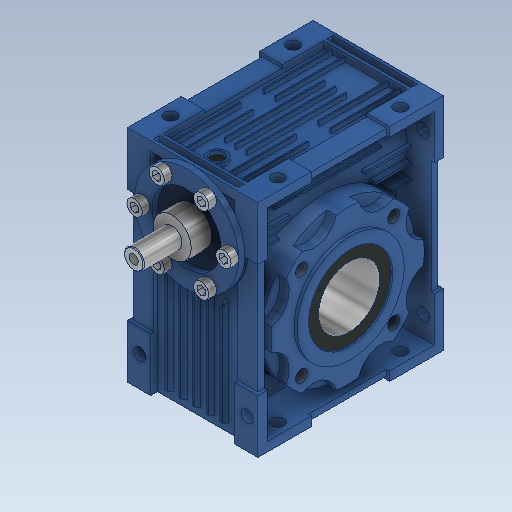
# Autodesk Inventor part: nmrv 50 casing
Saved by Autodesk Inventor 2020 (Build 240168000, 168)
## iProperties
Created: 2020-07-31
Part Number: nmrv 50 casing
Material: Generic
Document SubType Name: Modeling
Designer: Vikki
Density: 3.52796 g/cm^3
Appearance: Flaked Satin - Blue
Mass: 3500 g
Surface Area: 1630.31 cm^2
Volume: 992.076 cm^3
Author: Vikki
Autodesk Inventor part; units mm, degrees
sketch "Sketch1" plane through (0, 0, 0) normal (1, 0, 0) x (0, 1, 0)
  line L0 (-72, 60.5) -> (72, 60.5)
  line L1 (72, 60.5) -> (72, -60.5)
  line L2 (72, -60.5) -> (-72, -60.5)
  line L3 (-72, -60.5) -> (-72, 60.5)
  line L4 (-72, 60.5) -> (72, -60.5) construction
  line L5 (72, 60.5) -> (-72, -60.5) construction
  circle A0 centre (0, 0) radius 20
  dimension "d0" = 144
  dimension "d1" = 121
  dimension "d2" = 40
  constraints: 12 end point, 2 parallel, 1 centre point, 1 horizontal, 1 perpendicular, 1 vertical
  measures "d0" distance of L1.end L2.end
  measures "d1" distance of L0.end L1.end
  measures "d2" diameter of A0
extrude "Extrusion1" add sketch "Sketch1" along normal blind 85
ref_plane "Work Plane4" through (72.5, 0, 0) normal (1, 0, 0) x (0, 0, -1)
ref_plane "Work Plane5" through (85, 0, 0) normal (1, 0, 0) x (0, 0, -1)
sketch "Sketch10" plane through (0, 72, 60.5) normal (0, 1, 0) x (1, 0, 0)
  line L0 (0, 121) -> (0, 0) projected
  line L1 (0, 0) -> (85, 0) projected
  line L2 (85, 121) -> (85, 0) projected
  line L3 (0, 121) -> (85, 121) projected
  line L4 (0, 121) -> (0, 0) projected
  line L5 (0, 121) -> (85, 121) projected
  line L6 (0, 0) -> (85, 121)
  line L7 (0, 121) -> (85, 0)
  line L8 (77.5, 20.5) -> (7.5, 20.5)
  line L9 (7.5, 20.5) -> (7.5, 100.5)
  line L10 (7.5, 100.5) -> (77.5, 100.5)
  line L11 (77.5, 100.5) -> (77.5, 20.5)
  line L12 (77.5, 20.5) -> (7.5, 100.5) construction
  line L13 (7.5, 20.5) -> (77.5, 100.5) construction
  circle A0 centre (7.5, 20.5) radius 4.1
  circle A1 centre (7.5, 100.5) radius 4.1
  circle A2 centre (77.5, 100.5) radius 4.1
  circle A3 centre (77.5, 20.5) radius 4.1
  point P0 (0, 60.5)
  point P1 (42.5, 60.5)
  dimension "d60" = 70
  dimension "d61" = 80
  dimension "d62" = 8.2
  constraints: 16 end point, 4 centre point, 4 coincident, 3 equal radius, 3 midpoint, 2 parallel, 1 horizontal, 1 perpendicular
  measures "d60" distance of L9.end L10.end
  measures "d61" distance of L8.end L9.end
  measures "d62" diameter of A0
extrude "Extrusion10" cut sketch "Sketch10" against normal blind 10 contours A1 L9 L10 | L10 L9 A1 | A0 L9 L8 | L8 L9 A0 | A2 L11 L10 | L10 L11 A2 | A3 L11 L8 | L8 L11 A3
ref_plane "Work Plane6" through (0, 57, 60.5) normal (0, -1, 0) x (1, 0, 0)
sketch "Sketch14" plane through (0, 72, 60.5) normal (0, 1, 0) x (1, 0, 0)
  line L0 (0, 0) -> (85, 0) projected
  line L1 (0, 121) -> (85, 121) projected
  line L2 (0, 0) -> (85, 121)
  line L3 (0, 121) -> (0, 0) projected
  line L4 (0, 121) -> (85, 0)
  line L5 (70, -9.5) -> (15, -9.5)
  line L6 (15, -9.5) -> (15, 130.5)
  line L7 (15, 130.5) -> (70, 130.5)
  line L8 (70, 130.5) -> (70, -9.5)
  line L9 (70, -9.5) -> (15, 130.5) construction
  line L10 (15, -9.5) -> (70, 130.5) construction
  point P0 (0, 60.5)
  point P1 (42.5, 60.5)
  dimension "d74" = 140
  dimension "d75" = 55
  constraints: 16 end point, 3 midpoint, 2 parallel, 1 horizontal, 1 perpendicular
  measures "d74" distance of L5.end L6.end
  measures "d75" distance of L6.end L7.end
extrude "Extrusion13" cut sketch "Sketch14" against normal blind 5 contours L6 L2 L4 L8 L0 | L0 L8 L5 L6 | L6 L4 L2 | L4 L6 L1 L8 L2 | L2 L8 L4 | L6 L7 L8 L1
sketch "Sketch15" plane through (0, 67, 60.5) normal (0, 1, 0) x (1, 0, 0)
  line L0 (15, 0) -> (70, 0)
  line L1 (70, 0) -> (70, 2)
  line L2 (70, 2) -> (15, 2)
  line L3 (15, 2) -> (15, 0)
  line L4 (15, 6) -> (70, 6)
  line L5 (70, 6) -> (70, 8)
  line L6 (70, 8) -> (15, 8)
  line L7 (15, 8) -> (15, 6)
  point P0 (0, 60.5)
  dimension "d78" = 2
  dimension "d81" = 6
  constraints: 16 end point, 2 parallel, 1 coincident, 1 collinear, 1 horizontal, 1 perpendicular, 1 vertical, 7 other
  measures "d78" distance between parallel lines of L0 L2
  measures "d81" distance of L0.end L4.end
extrude "Extrusion14" add sketch "Sketch15" along normal blind 5
ref_plane "Work Plane1" through (0, -72, 0) normal (0, 0, 1) x (1, 0, 0)
mirror "Mirror1" about plane through (0, -72, 0) normal (0, 0, 1) of "Extrusion14"
sketch "Sketch16" plane through (0, 67, 60.5) normal (0, 1, 0) x (1, 0, 0)
  circle A0 centre (42.5, 16) radius 6
  line L0 (15, 8) -> (15, 113) projected
  line L1 (70, 8) -> (15, 8) projected
  circle A1 centre (42.5, 16) radius 4.5
  point P0 (0, 60.5)
  dimension "d88" = 27.5
  dimension "d89" = 8
  dimension "d90" = 12
  dimension "d91" = 1.5
  constraints: 2 centre point
  measures "d88" distance from line of A0.centre L0
  measures "d89" distance from line of L1 A0.centre
  measures "d90" diameter of A0
  measures "d91" radial gap between concentric circles of A0 A1
extrude "Extrusion15" add sketch "Sketch16" along normal blind 2
sketch "Sketch17" plane through (0, 67, 60.5) normal (0, 1, 0) x (1, 0, 0)
  line L0 (35, 28.020714) -> (36, 28.020714)
  line L1 (36, 28.020714) -> (36, 74)
  line L2 (36, 74) -> (35, 74)
  line L3 (35, 74) -> (35, 28.020714)
  line L4 (15, 8) -> (15, 113)
  line L5 (49, 28.020714) -> (50, 28.020714)
  line L6 (50, 28.020714) -> (50, 68.020714)
  line L7 (50, 68.020714) -> (49, 68.020714)
  line L8 (49, 68.020714) -> (49, 28.020714)
  line L9 (70, 113) -> (70, 8)
  line L10 (42, 28.020714) -> (43, 28.020714)
  line L11 (43, 28.020714) -> (43, 74)
  line L12 (43, 74) -> (42, 74)
  line L13 (42, 74) -> (42, 28.020714)
  point P0 (0, 60.5)
  dimension "d94" = 20
  dimension "d95" = 1
  dimension "d96" = 1
  dimension "d97" = 20
  dimension "d98" = 1
  dimension "d99" = 6
  dimension "d100" = 40
  constraints: 24 end point, 6 parallel, 3 collinear, 3 horizontal, 3 perpendicular
  measures "d94" distance between parallel lines of L3 L4
  measures "d95" distance of L0.start L0.end
  measures "d96" distance of L5.start L5.end
  measures "d97" distance between parallel lines of L9 L6
  measures "d98" distance of L10.start L10.end
  measures "d99" distance between parallel lines of L13 L1
  measures "d100" distance of L5.end L6.end
extrude "Extrusion16" add sketch "Sketch17" along normal blind 3
sketch "Sketch18" plane through (0, 67, 60.5) normal (0, 1, 0) x (1, 0, 0)
  line L0 (20, 8) -> (21, 8)
  line L1 (21, 8) -> (21, 53)
  line L2 (21, 53) -> (20, 53)
  line L3 (20, 53) -> (20, 8)
  line L4 (15, 8) -> (70, 8)
  line L5 (28, 8) -> (29, 8)
  line L6 (29, 8) -> (29, 53)
  line L7 (29, 53) -> (28, 53)
  line L8 (28, 53) -> (28, 8)
  line L9 (42, 74) -> (42, 28.020714)
  line L10 (43, 28.020714) -> (43, 74)
  line L11 (42.5, 29) -> (42.5, 35)
  line L12 (42.5, 35) -> (42.5, 36)
  line L13 (42.5, 36) -> (42.5, 26)
  line L14 (65, 8) -> (64, 8)
  line L15 (64, 8) -> (64, 53)
  line L16 (64, 53) -> (65, 53)
  line L17 (65, 53) -> (65, 8)
  line L18 (57, 8) -> (56, 8)
  line L19 (56, 8) -> (56, 53)
  line L20 (56, 53) -> (57, 53)
  line L21 (57, 53) -> (57, 8)
  point P0 (0, 60.5)
  point P1 (64, 8)
  point P2 (65, 8)
  point P3 (57, 8)
  point P4 (28, 8)
  dimension "d103" = 1
  dimension "d104" = 45
  dimension "d107" = 8
  dimension "d112" = 0.5
  constraints: 38 end point, 8 symmetric about line, 3 parallel, 2 collinear, 2 horizontal, 1 perpendicular, 7 other
  measures "d103" distance of L0.start L0.end
  measures "d104" distance of L0.end L1.end
  measures "d107" distance of L0.start L5.start
  measures "d112" distance between parallel lines of L9 L13
extrude "Extrusion17" add sketch "Sketch18" along normal blind 3
mirror "Mirror2" about plane through (0, -72, 0) normal (0, 0, 1) of "Extrusion16", "Extrusion17"
ref_plane "Work Plane2" through (0, 0, 60.5) normal (0, 1, 0) x (1, 0, 0)
mirror "Mirror3" about plane through (0, 0, 60.5) normal (0, 1, 0) of "Extrusion16", "Extrusion17", "Mirror2", "Extrusion14", "Mirror1", "Extrusion13", "Extrusion10"
ref_plane "Work Plane3" through (42.5, 0, 0) normal (1, 0, 0) x (0, 0, -1)
sketch "Sketch22" plane through (85, 0, 0) normal (1, 0, 0) x (0, 0, -1)
  circle A0 centre (0, 0) radius 20 projected
extrude "Extrusion18" add sketch "Sketch22" against normal up to surface (85 mm away)
sketch "Sketch23" plane through (85, 0, 0) normal (1, 0, 0) x (0, 0, -1)
  circle A0 centre (0, -12) radius 20
  line L0 (60.5, 72) -> (-60.5, 72) projected
  point P0 (0, 0)
  dimension "d130" = 84
  dimension "d131" = 40
  constraints: 1 centre point, 1 vertical alignment
  measures "d130" distance from line of A0.centre L0
  measures "d131" diameter of A0
extrude "Extrusion19" cut sketch "Sketch23" against normal up to surface (85 mm away)
sketch "Sketch24" plane through (85, 0, 0) normal (1, 0, 0) x (0, 0, -1)
  circle A0 centre (0, -12) radius 20 projected
  line L0 (60.5, 72) -> (-60.5, 72) projected
  line L1 (-60.5, 72) -> (-60.5, -72) projected
  line L2 (-60.5, -72) -> (60.5, -72) projected
  line L3 (60.5, -72) -> (60.5, 72) projected
  circle A1 centre (0, -12) radius 50
  line L4 (-54.5, 66) -> (54.5, 66)
  line L5 (54.5, 66) -> (54.5, -66)
  line L6 (54.5, -66) -> (-54.5, -66)
  line L7 (-54.5, -66) -> (-54.5, 66)
  point P0 (0, 0)
  dimension "d134" = 100
  dimension "d135" = 6
  constraints: 8 end point, 1 centre point, 1 coincident, 3 other
  measures "d134" diameter of A1
  measures "d135" distance between parallel lines of L4 L0
extrude "Extrusion20" cut sketch "Sketch24" against normal blind 25 contours L4 L5 L6 L7
sketch "Sketch25" plane through (85, -12, 0) normal (1, 0, 0) x (0, 0, -1)
  circle A0 centre (0, 0) radius 20
  circle A1 centre (0, 0) radius 50
  circle A2 centre (0, 0) radius 20
  line L0 (0, 0) -> (25.019992, 25.019992) construction
  line L1 (0, 0) -> (34, 0)
  circle A3 centre (0, 0) radius 42.5
  line L2 (0, 0) -> (53.123073, 22.004297) construction
  circle A4 centre (53.123073, 22.004297) radius 15
  circle A5 centre (22.004297, 53.123073) radius 15
  circle A6 centre (-22.004297, 53.123073) radius 15
  circle A7 centre (-53.123073, 22.004297) radius 15
  circle A8 centre (-53.123073, -22.004297) radius 15
  circle A9 centre (-22.004297, -53.123073) radius 15
  circle A10 centre (22.004297, -53.123073) radius 15
  circle A11 centre (53.123073, -22.004297) radius 15
  point P0 (0, 12)
  point P1 (-40.23675, 29.681711)
  point P2 (-49.439818, 7.46354)
  point P3 (-49.439818, -7.46354)
  point P4 (-40.23675, -29.681711)
  point P5 (-29.681711, -40.23675)
  point P6 (-7.46354, -49.439818)
  point P7 (7.46354, -49.439818)
  point P8 (29.681711, -40.23675)
  point P9 (40.23675, -29.681711)
  point P10 (49.439818, -7.46354)
  point P11 (49.439818, 7.46354)
  point P12 (40.23675, 29.681711)
  point P13 (-7.46354, 49.439818)
  point P14 (-29.681711, 40.23675)
  point P15 (29.681711, 40.23675)
  point P16 (7.46354, 49.439818)
  dimension "d138" = 45
  dimension "d139" = 85
  dimension "d140" = 22.5
  dimension "d141" = 30
  dimension "d144" = 360
  constraints: 9 centre point, 6 end point, 2 coincident, 1 horizontal, 1 tangent, 17 other
  measures "d138" angle of L1 L0
  measures "d139" diameter of A3
  measures "d140" angle of L1 L2
  measures "d141" diameter of A4
extrude "Extrusion21" cut sketch "Sketch25" against normal blind 8 contours A4 A1 | A1 A11 | A5 A1 | A1 A10 | A6 A1 | A9 A1 | A7 A1 | A8 A1 picked at (43.783416, 18.135685) picked at (43.783416, -18.135685) picked at (18.135685, 43.783416) picked at (18.135685, -43.783416) picked at (-18.135685, 43.783416) picked at (-18.135685, -43.783416) picked at (-43.783416, 18.135685) picked at (-43.783416, -18.135685)
sketch "Sketch26" plane through (85, 0, 0) normal (1, 0, 0) x (0, 0, -1)
  circle A0 centre (0, -12) radius 20
  circle A1 centre (0, -12) radius 35
  arc A2 (49.439818, -19.46354) -> (49.439818, -4.53646) centre (0, -12) ccw
  arc A3 (40.23675, -41.681711) -> (49.439818, -19.46354) centre (0, -12) ccw
  arc A4 (29.681711, -52.23675) -> (40.23675, -41.681711) centre (0, -12) ccw
  arc A5 (7.46354, -61.439818) -> (29.681711, -52.23675) centre (0, -12) ccw
  arc A6 (-7.46354, -61.439818) -> (7.46354, -61.439818) centre (0, -12) ccw
  arc A7 (-29.681711, -52.23675) -> (-7.46354, -61.439818) centre (0, -12) ccw
  arc A8 (-40.23675, -41.681711) -> (-29.681711, -52.23675) centre (0, -12) ccw
  arc A9 (-49.439818, -19.46354) -> (-40.23675, -41.681711) centre (0, -12) ccw
  arc A10 (-49.439818, -4.53646) -> (-49.439818, -19.46354) centre (0, -12) ccw
  arc A11 (-40.23675, 17.681711) -> (-49.439818, -4.53646) centre (0, -12) ccw
  arc A12 (-29.681711, 28.23675) -> (-40.23675, 17.681711) centre (0, -12) ccw
  arc A13 (-7.46354, 37.439818) -> (-29.681711, 28.23675) centre (0, -12) ccw
  arc A14 (7.46354, 37.439818) -> (-7.46354, 37.439818) centre (0, -12) ccw
  arc A15 (29.681711, 28.23675) -> (7.46354, 37.439818) centre (0, -12) ccw
  arc A16 (40.23675, 17.681711) -> (29.681711, 28.23675) centre (0, -12) ccw
  arc A17 (49.439818, -4.53646) -> (40.23675, 17.681711) centre (0, -12) ccw
  circle A18 centre (0, -12) radius 50
  point P0 (0, 0)
  point P1 (49.439818, -4.53646)
  point P2 (29.681711, 28.23675)
  point P3 (-7.46354, 37.439818)
  point P4 (-49.439818, -19.46354)
  point P5 (7.46354, -61.439818)
  dimension "d148" = 70
  constraints: 1 centre point, 1 coincident
  measures "d148" diameter of A1
extrude "Extrusion22" cut sketch "Sketch26" against normal blind 2 contours A3 A4 A5 A6 A7 A8 A9 A10 A11 A12 A13 A14 A15 A16 A17 A2
sketch "Sketch27" plane through (85, -12, 0) normal (1, 0, 0) x (0, 0, -1)
  circle A0 centre (0, 0) radius 20 projected
  circle A1 centre (0, 0) radius 27.5
  point P0 (0, 12)
  dimension "d151" = 55
  constraints: 1 centre point, 1 coincident
  measures "d151" diameter of A1
extrude "Extrusion23" cut sketch "Sketch27" against normal blind 1
sketch "Sketch28" plane through (83, 0, 0) normal (1, 0, 0) x (0, 0, -1)
  circle A0 centre (0, -12) radius 20
  circle A1 centre (30.052038, 18.052038) radius 4
  circle A2 centre (0, -12) radius 42.5
  line L0 (0, -12) -> (13, -12)
  line L1 (0, -12) -> (30.052038, 18.052038) construction
  line L2 (0, -12) -> (-30.052038, 18.052038) construction
  circle A3 centre (-30.052038, 18.052038) radius 4
  line L3 (0, -12) -> (-30.052038, -42.052038) construction
  circle A4 centre (-30.052038, -42.052038) radius 4
  line L4 (0, -12) -> (30.052038, -42.052038) construction
  circle A5 centre (30.052038, -42.052038) radius 4
  point P0 (0, 0)
  dimension "d154" = 85
  dimension "d155" = 45
  dimension "d156" = 8
  dimension "d159" = 360
  constraints: 10 end point, 4 centre point, 1 coincident, 1 horizontal, 20 other
  measures "d155" angle of L0 L1
  measures "d156" diameter of A1
extrude "Extrusion24" cut sketch "Sketch28" against normal blind 10 contours A1 A2 | A2 A1 | A3 A2 | A2 A3 | A5 A2 | A2 A5 | A4 A2 | A2 A4
thread "Thread7" size "M8x1.25" class "6H" standard "ANSI Metric M Profile" length 60
thread "Thread8" size "M8x1.25" class "6H" standard "ANSI Metric M Profile" length 60
thread "Thread9" size "M8x1.25" class "6H" standard "ANSI Metric M Profile" length 60
thread "Thread10" size "M8x1.25" class "6H" standard "ANSI Metric M Profile" length 60
sketch "Sketch29" plane through (60, 0, 0) normal (1, 0, 0) x (0, 0, -1)
  line L0 (-35, 58) -> (0, 58)
  line L1 (0, 58) -> (0, 56.5)
  line L2 (0, 56.5) -> (-35, 56.5)
  line L3 (-35, 56.5) -> (-35, 58)
  line L4 (-54.5, 66) -> (54.5, 66) projected
  line L5 (-35, 49) -> (0, 49)
  line L6 (0, 49) -> (0, 47.5)
  line L7 (0, 47.5) -> (-35, 47.5)
  line L8 (-35, 47.5) -> (-35, 49)
  line L9 (-54.5, -66) -> (-54.5, 66) projected
  line L10 (-54.5, 39.5) -> (-24.5, 39.5)
  line L11 (-24.5, 39.5) -> (-24.5, 38)
  line L12 (-24.5, 38) -> (-54.5, 38)
  line L13 (-54.5, 38) -> (-54.5, 39.5)
  line L14 (-54.5, -66) -> (-54.5, 66) projected
  line L15 (-54.5, 30) -> (-31.5, 30)
  line L16 (-31.5, 30) -> (-31.5, 28.5)
  line L17 (-31.5, 28.5) -> (-54.5, 28.5)
  line L18 (-54.5, 28.5) -> (-54.5, 30)
  line L19 (-54.5, 20.5) -> (-41.5, 20.5)
  line L20 (-41.5, 20.5) -> (-41.5, 19)
  line L21 (-41.5, 19) -> (-54.5, 19)
  line L22 (-54.5, 19) -> (-54.5, 20.5)
  line L23 (0, 49) -> (0, 56.5)
  line L24 (35, 58) -> (0, 58)
  line L25 (0, 56.5) -> (35, 56.5)
  line L26 (35, 56.5) -> (35, 58)
  line L27 (35, 49) -> (0, 49)
  line L28 (0, 47.5) -> (35, 47.5)
  line L29 (35, 47.5) -> (35, 49)
  line L30 (54.5, 39.5) -> (24.5, 39.5)
  line L31 (24.5, 39.5) -> (24.5, 38)
  line L32 (24.5, 38) -> (54.5, 38)
  line L33 (54.5, 38) -> (54.5, 39.5)
  line L34 (54.5, 30) -> (31.5, 30)
  line L35 (31.5, 30) -> (31.5, 28.5)
  line L36 (31.5, 28.5) -> (54.5, 28.5)
  line L37 (54.5, 28.5) -> (54.5, 30)
  line L38 (54.5, 20.5) -> (41.5, 20.5)
  line L39 (41.5, 20.5) -> (41.5, 19)
  line L40 (41.5, 19) -> (54.5, 19)
  line L41 (54.5, 19) -> (54.5, 20.5)
  point P0 (0, 0)
  dimension "d171" = 1.5
  dimension "d172" = 8
  dimension "d173" = 35
  dimension "d176" = 9
  dimension "d181" = 30
  dimension "d182" = 8
  dimension "d183" = 8
  dimension "d184" = 8
  dimension "d185" = 23
  dimension "d186" = 13
  constraints: 78 end point, 16 symmetric about line, 11 parallel, 4 horizontal, 4 perpendicular, 3 point on line, 2 vertical, 1 collinear, 1 vertical alignment, 7 other
  measures "d171" distance of L2.end L0.start
  measures "d172" distance between parallel lines of L0 L4
  measures "d173" distance of L0.start L0.end
  measures "d176" distance of L0.start L5.start
  measures "d181" distance of L10.start L10.end
  measures "d182" distance between parallel lines of L10 L7
  measures "d183" distance between parallel lines of L15 L12
  measures "d184" distance between parallel lines of L19 L17
  measures "d185" distance of L15.start L15.end
  measures "d186" distance of L19.start L19.end
extrude "Extrusion25" add sketch "Sketch29" along normal blind 10
mirror "Mirror5" about plane through (42.5, 0, 0) normal (1, 0, 0) of "Extrusion20", "Extrusion21", "Extrusion23", "Extrusion22", "Extrusion24", "Extrusion25"
sketch "Sketch31" plane through (0, -72, 60.5) normal (0, 0, 1) x (1, 0, 0)
  circle A0 centre (42.5, 110) radius 29
  line L0 (1, 80) -> (1, 40)
  line L1 (1, 60) -> (49, 60)
  line L2 (85, 144) -> (85, 0)
  line L3 (42.5, 110) -> (57, 135.114737)
  line L4 (0, 0) -> (85, 0)
  circle A1 centre (57, 135.114737) radius 3
  circle A2 centre (28, 135.114737) radius 3
  circle A3 centre (13.5, 110) radius 3
  circle A4 centre (28, 84.885263) radius 3
  circle A5 centre (57, 84.885263) radius 3
  circle A6 centre (71.5, 110) radius 3
  circle A7 centre (78, 20) radius 4.1
  circle A8 centre (8, 20) radius 4.1
  point P0 (0, 72)
  dimension "d192" = 58
  dimension "d189" = 20
  dimension "d190" = 50
  dimension "d191" = 42.5
  dimension "d193" = 60
  dimension "d194" = 6
  dimension "d197" = 360
  dimension "d202" = 70
  dimension "d203" = 8.2
  dimension "d204" = 20
  constraints: 8 centre point, 4 end point, 1 coincident, 1 equal radius, 1 horizontal, 1 horizontal alignment, 1 midpoint, 16 other
  measures "d189" distance from line of L1 L0.start
  measures "d190" distance from line of L1 L3.start
  measures "d191" distance from line of L2 L3.start
  measures "d193" angle of L4 L3
  measures "d194" diameter of A1
  measures "d202" distance of A8.centre A7.centre
  measures "d203" diameter of A7
  measures "d204" distance from line of L4 A8.centre
extrude "Extrusion26" cut sketch "Sketch31" against normal blind 8 contours A0 A6 | A0 A6 | A1 L3 A0 | A0 A1 | A5 A0 | A0 A5 | L3 A1 A0 | A4 A0 | A0 A4 | A2 A0 | A0 A2 | A3 A0 | A0 A3 | A7 | A8
sketch "Sketch32" plane through (0, -72, 60.5) normal (0, 0, 1) x (1, 0, 0)
  circle A0 centre (42.5, 110) radius 34
  circle A1 centre (28, 135.114737) radius 3
  circle A2 centre (71.5, 110) radius 3
  circle A3 centre (57, 84.885263) radius 3
  circle A4 centre (78, 20) radius 4.1
  circle A5 centre (13.5, 110) radius 3
  circle A6 centre (57, 135.114737) radius 3
  circle A7 centre (28, 84.885263) radius 3
  circle A8 centre (8, 20) radius 4.1
  line L0 (0, 0) -> (85, 0)
  line L1 (85, 144) -> (85, 0)
  line L2 (0, 144) -> (85, 144)
  line L3 (0, 144) -> (0, 0)
  circle A9 centre (42.5, 110) radius 22.5
  point P0 (0, 72)
  dimension "d201" = 68
  dimension "d205" = 45
  constraints: 2 centre point, 2 coincident
  measures "d201" diameter of A0
  measures "d205" diameter of A9
extrude "Extrusion27" add sketch "Sketch32" along normal blind 4 contours A0
sketch "Sketch33" plane through (42.5, 38, 60.5) normal (0, 0, 1) x (1, 0, 0)
  circle A0 centre (0, 0) radius 22.5 projected
  circle A1 centre (0, 0) radius 12.5
  point P0 (-42.5, -38)
  dimension "d208" = 25
  constraints: 1 centre point, 1 coincident
  measures "d208" diameter of A1
extrude "Extrusion28" add sketch "Sketch33" along normal blind 13.5 contours A1
sketch "Sketch34" plane through (42.5, 38, 74) normal (0, 0, 1) x (1, 0, 0)
  circle A0 centre (0, 0) radius 12.5 projected
  circle A1 centre (0, 0) radius 6.5
  point P0 (-42.5, -38)
  dimension "d211" = 13
  constraints: 1 centre point, 1 coincident
  measures "d211" diameter of A1
extrude "Extrusion29" add sketch "Sketch34" along normal blind 25 contours A1
sketch "Sketch35" plane through (42.5, 38, 64.5) normal (0, 0, 1) x (1, 0, 0)
  circle A0 centre (29, 0) radius 3 projected
  circle A1 centre (29, 0) radius 5
  point P0 (-42.5, -38)
  constraints: 1 centre point, 1 coincident
extrude "Extrusion30" add sketch "Sketch35" along normal blind 5 contours A0 | A1
sketch "Sketch36" plane through (71.5, 38, 69.5) normal (0, 0, 1) x (1, 0, 0)
  arc A0 (-3, 0) -> (-2.598076, 1.5) centre (0, 0) ccw
  circle A1 centre (0, 0) radius 3
  circle A2 centre (0, 0) radius 5
  circle A3 centre (0, 0) radius 3
  line L0 (2.598076, 1.5) -> (2.598076, -1.5)
  line L1 (2.598076, -1.5) -> (0, -3)
  line L2 (0, -3) -> (-2.598076, -1.5)
  line L3 (-2.598076, -1.5) -> (-2.598076, 1.5)
  line L4 (-2.598076, 1.5) -> (0, 3)
  line L5 (0, 3) -> (2.598076, 1.5)
  point P0 (-71.5, -38)
  point P1 (5, 0)
  constraints: 12 end point, 2 coincident, 1 centre point, 1 horizontal alignment, 1 point on circle, 13 other
extrude "Extrusion31" cut sketch "Sketch36" against normal blind 4 contours L3 L4 L5 L0 L1 L2
pattern_circular "Circular Pattern2" count 6 over 360 about axis through (42.5, 38, 74) along (0, 0, 1) of "Extrusion30", "Extrusion31"
sketch "Sketch37" plane through (0, -72, 60.5) normal (0, 0, 1) x (1, 0, 0)
  line L0 (70, 139) -> (70, 144) projected
  line L1 (15, 144) -> (15, 139) projected
  line L2 (15, 139) -> (15, 0)
  line L3 (0, 0) -> (85, 0) projected
  line L4 (70, 139) -> (70, 0)
  circle A0 centre (42.5, 110) radius 34 projected
  line L5 (70, 139) -> (15, 139) projected
  line L6 (15, 138) -> (70, 138)
  point P0 (0, 72)
  point P1 (42.5, 144)
  point P2 (70, 90.006251)
  point P3 (15, 90.006251)
  point P4 (61.787302, 138)
  point P5 (70, 129.993749)
  point P6 (23.212698, 138)
  point P7 (15, 129.993749)
  dimension "d221" = 90
  dimension "d222" = 1
  constraints: 6 end point, 4 point on line, 1 parallel, 1 perpendicular, 1 other
  measures "d221" angle of L2 L3
  measures "d222" distance between parallel lines of L5 L6
extrude "Extrusion32" cut sketch "Sketch37" against normal blind 4.5 contours L6 A0 L2 | A0 L4 L3 L2 | L6 L4 A0
sketch "Sketch38" plane through (85, -72, 60.5) normal (0, 0, 1) x (1, 0, 0)
  arc A0 (-15, 90.006251) -> (-15, 129.993749) centre (-42.5, 110) ccw
  arc A1 (-8.5, 110) -> (-25.5, 139.444864) centre (-42.5, 110) ccw
  arc A2 (-25.5, 80.555136) -> (-8.5, 110) centre (-42.5, 110) ccw
  arc A3 (-59.5, 80.555136) -> (-25.5, 80.555136) centre (-42.5, 110) ccw
  arc A4 (-76.5, 110) -> (-59.5, 80.555136) centre (-42.5, 110) ccw
  arc A5 (-59.5, 139.444864) -> (-76.5, 110) centre (-42.5, 110) ccw
  arc A6 (-25.5, 139.444864) -> (-59.5, 139.444864) centre (-42.5, 110) ccw
  arc A7 (-23.212698, 138) -> (-42.5, 144) centre (-42.5, 110) ccw
  arc A8 (-42.5, 144) -> (-61.787302, 138) centre (-42.5, 110) ccw
  arc A9 (-61.787302, 138) -> (-70, 129.993749) centre (-42.5, 110) ccw
  arc A10 (-70, 129.993749) -> (-70, 90.006251) centre (-42.5, 110) ccw
  arc A11 (-70, 90.006251) -> (-15, 90.006251) centre (-42.5, 110) ccw
  arc A12 (-15, 90.006251) -> (-15, 129.993749) centre (-42.5, 110) ccw
  arc A13 (-15, 129.993749) -> (-23.212698, 138) centre (-42.5, 110) ccw
  point P0 (-85, 72)
extrude "Extrusion33" cut sketch "Sketch38" against normal blind 4
sketch "Sketch39" plane through (0, -72, 56) normal (0, 0, 1) x (1, 0, 0)
  circle A0 centre (57, 84.885263) radius 3
  circle A1 centre (57, 135.114737) radius 3
  arc A2 (68.5, 110) -> (68.901924, 111.5) centre (71.5, 110) ccw
  arc A3 (68.5, 110) -> (68.901924, 111.5) centre (71.5, 110) ccw
  arc A4 (68.901924, 111.5) -> (68.5, 110) centre (71.5, 110) ccw
  circle A5 centre (71.5, 110) radius 3
  circle A6 centre (28, 84.885263) radius 3
  circle A7 centre (28, 84.885263) radius 3
  arc A8 (16.5, 110) -> (16.098076, 111.5) centre (13.5, 110) ccw
  arc A9 (16.098076, 111.5) -> (16.5, 110) centre (13.5, 110) ccw
  circle A10 centre (13.5, 110) radius 3
  circle A11 centre (28, 135.114737) radius 3
  circle A12 centre (28, 135.114737) radius 3
  point P0 (0, 72)
  point P1 (60, 84.885263)
  point P2 (60, 135.114737)
  point P3 (25, 84.885263)
  point P4 (25, 84.885263)
  point P5 (25, 135.114737)
  point P6 (25, 135.114737)
  constraints: 4 horizontal alignment
extrude "Extrusion34" add sketch "Sketch39" along normal blind 4
sketch "Sketch40" plane through (0, 67, 60.5) normal (0, 1, 0) x (1, 0, 0)
  line L0 (24.751761, 2) -> (24.751761, 4)
  line L1 (24.751761, 4) -> (60.248239, 4)
  line L2 (60.248239, 4) -> (60.248239, 2)
  line L3 (60.248239, 2) -> (70, 2)
  line L4 (70, 6) -> (70, 2)
  line L5 (70, 6) -> (15, 6)
  line L6 (15, 2) -> (15, 6)
  line L7 (15, 2) -> (24.751761, 2)
  line L8 (70, 2) -> (42.5, 2)
  line L9 (42.5, 2) -> (15, 2)
  point P0 (0, 60.5)
extrude "Extrusion35" add sketch "Sketch40" along normal blind 1
sketch "Sketch41" plane through (15, -67, 54.5) normal (0, 0, 1) x (1, 0, 0)
  line L0 (0, 0) -> (55, 0) projected
  line L1 (0, -5) -> (0, 0) projected
  line L2 (0, -5) -> (55, -5) projected
  line L3 (55, 0) -> (55, -5) projected
  point P0 (-15, 67)
extrude "Extrusion36" add sketch "Sketch41" along normal up to surface (1.5 mm away)
sketch "Sketch42" plane through (0, -72, 56) normal (0, 0, 1) x (1, 0, 0)
  line L0 (23.75, 75) -> (25.25, 75)
  line L1 (25.25, 75) -> (25.25, 5)
  line L2 (25.25, 5) -> (23.75, 5)
  line L3 (23.75, 5) -> (23.75, 75)
  line L4 (70, 0) -> (15, 0)
  line L5 (15, 0) -> (15, 90.006251)
  line L6 (32.75, 75) -> (34.25, 75)
  line L7 (34.25, 75) -> (34.25, 5)
  line L8 (34.25, 5) -> (32.75, 5)
  line L9 (32.75, 5) -> (32.75, 75)
  line L10 (41.75, 75) -> (43.25, 75)
  line L11 (43.25, 75) -> (43.25, 5)
  line L12 (43.25, 5) -> (41.75, 5)
  line L13 (41.75, 5) -> (41.75, 75)
  line L14 (50.75, 75) -> (52.25, 75)
  line L15 (52.25, 75) -> (52.25, 5)
  line L16 (52.25, 5) -> (50.75, 5)
  line L17 (50.75, 5) -> (50.75, 75)
  line L18 (59.75, 75) -> (61.25, 75)
  line L19 (61.25, 75) -> (61.25, 5)
  line L20 (61.25, 5) -> (59.75, 5)
  line L21 (59.75, 5) -> (59.75, 75)
  point P0 (0, 72)
  dimension "d233" = 1.5
  dimension "d234" = 70
  dimension "d235" = 5
  dimension "d236" = 8.75
  dimension "d239" = 9
  constraints: 40 end point, 2 horizontal, 2 parallel, 1 perpendicular, 32 other
  measures "d233" distance of L1.end L2.end
  measures "d234" distance of L2.end L0.start
  measures "d235" distance from line of L1.end L4
  measures "d236" distance between parallel lines of L5 L3
  measures "d239" distance of L0.start L6.start
extrude "Extrusion37" add sketch "Sketch42" along normal blind 4
sketch "Sketch43" plane through (23.75, -67, 56) normal (-1, 0, 0) x (0, 0, 1)
  line L0 (0, 0) -> (0, 70)
  line L1 (0, 0) -> (4, 0)
  line L2 (4, 70) -> (4, 0)
  line L3 (0, 70) -> (4, 70)
  line L4 (0, 69.893427) -> (4, 67.584026)
  line L5 (4, 70) -> (4, 0)
  line L6 (0, 0) -> (0, 70)
  line L7 (0, 0) -> (4, 2.309401)
  point P0 (-56, 67)
  dimension "d246" = 30
  dimension "d247" = 60
  constraints: 4 end point, 3 point on line
  measures "d246" angle of L3 L4
  measures "d247" angle of L7 L0
extrude "Extrusion38" cut sketch "Sketch43" against normal up to surface (37.5 mm away) contours L7 L2 L1 | L0 L3 L2 L4
sketch "Sketch44" plane through (0, -72, 56) normal (0, 0, 1) x (1, 0, 0)
  arc A0 (70, 90.006251) -> (61.787302, 138) centre (42.5, 110) ccw
  circle A1 centre (42.5, 110) radius 6.5
  circle A2 centre (42.5, 110) radius 25
  point P0 (0, 72)
  dimension "d250" = 50
  constraints: 1 centre point, 1 coincident
  measures "d250" diameter of A2
extrude "Extrusion39" add sketch "Sketch44" against normal up to surface (110.5 mm away) contours A1 | A2
sketch "Sketch45" plane through (42.5, 38, 99) normal (0, 0, 1) x (1, 0, 0)
  circle A0 centre (0, 0) radius 6.5 projected
  circle A1 centre (0, 0) radius 3
  point P0 (-42.5, -38)
  dimension "d253" = 6
  constraints: 1 centre point, 1 coincident
  measures "d253" diameter of A1
extrude "Extrusion40" cut sketch "Sketch45" against normal blind 10 contours A1
sketch "Sketch46" plane through (85, -72, 60.5) normal (0, 0, 1) x (1, 0, 0)
  line L0 (-117, 109) -> (40, 109)
  line L1 (40, 109) -> (40, 35)
  line L2 (40, 35) -> (-117, 35)
  line L3 (-117, 35) -> (-117, 109)
  circle A0 centre (-7, 20) radius 4.1
  line L4 (-85, 144) -> (-42.5, 144)
  circle A1 centre (-57, 84.885263) radius 3
  circle A2 centre (-57, 84.885263) radius 3
  circle A3 centre (-71.5, 110) radius 3
  circle A4 centre (-28, 84.885263) radius 3
  circle A5 centre (-13.5, 110) radius 3
  circle A6 centre (-28, 135.114737) radius 3
  circle A7 centre (-57, 135.114737) radius 3
  line L5 (-25.25, 7.309401) -> (-23.75, 7.309401)
  line L6 (-23.75, 7.309401) -> (-23.75, 72.584026)
  line L7 (-23.75, 72.584026) -> (-25.25, 72.584026)
  line L8 (-25.25, 72.584026) -> (-25.25, 7.309401)
  line L9 (-34.25, 7.309401) -> (-32.75, 7.309401)
  line L10 (-32.75, 7.309401) -> (-32.75, 72.584026)
  line L11 (-32.75, 72.584026) -> (-34.25, 72.584026)
  line L12 (-34.25, 72.584026) -> (-34.25, 7.309401)
  line L13 (-2, 30.318289) -> (-2, 19.76325)
  line L14 (-43.25, 7.309401) -> (-41.75, 7.309401)
  line L15 (-41.75, 7.309401) -> (-41.75, 72.584026)
  line L16 (-41.75, 72.584026) -> (-43.25, 72.584026)
  line L17 (-43.25, 72.584026) -> (-43.25, 7.309401)
  line L18 (-52.25, 7.309401) -> (-50.75, 7.309401)
  line L19 (-50.75, 7.309401) -> (-50.75, 72.584026)
  line L20 (-50.75, 72.584026) -> (-52.25, 72.584026)
  line L21 (-52.25, 72.584026) -> (-52.25, 7.309401)
  line L22 (-1, 40) -> (-84, 40)
  line L23 (-61.25, 7.309401) -> (-59.75, 7.309401)
  line L24 (-59.75, 7.309401) -> (-59.75, 72.584026)
  line L25 (-59.75, 72.584026) -> (-61.25, 72.584026)
  line L26 (-61.25, 72.584026) -> (-61.25, 7.309401)
  point P0 (-85, 72)
  point P1 (-61.25, 35)
  point P2 (-59.75, 40)
  point P3 (-52.25, 40)
  point P4 (-50.75, 40)
  point P5 (-43.25, 40)
  point P6 (-41.75, 40)
  point P7 (-34.25, 40)
  point P8 (-32.75, 40)
  point P9 (-25.25, 40)
  point P10 (-23.75, 35)
  dimension "d256" = 15
  dimension "d257" = 35
  constraints: 8 end point, 2 parallel, 1 horizontal, 1 perpendicular
  measures "d256" distance from line of A0.centre L2
  measures "d257" distance between parallel lines of L0 L4
extrude "Extrusion41" cut sketch "Sketch46" against normal blind 2 contours L0 A3 A5 L1 L2 L6 L7 L8 L22 L10 L11 L12 L15 L16 L17 L19 L20 L21 L24 L25 L26 L3
sketch "Sketch47" plane through (0, -72, -60.5) normal (0, 0, -1) x (-1, 0, 0)
  line L0 (-21, 2) -> (-21, 5)
  line L1 (-59.75, 5) -> (-59.75, 74.893427)
  line L2 (-59.75, 74.893427) -> (-61.25, 74.893427)
  line L3 (-61.25, 74.893427) -> (-61.25, 5)
  line L4 (-61.25, 5) -> (-59.75, 5)
  line L5 (-52.25, 5) -> (-50.75, 5)
  line L6 (-50.75, 5) -> (-50.75, 74.893427)
  line L7 (-50.75, 74.893427) -> (-52.25, 74.893427)
  line L8 (-52.25, 74.893427) -> (-52.25, 5)
  line L9 (-43.25, 5) -> (-41.75, 5)
  line L10 (-41.75, 5) -> (-41.75, 74.893427)
  line L11 (-41.75, 74.893427) -> (-43.25, 74.893427)
  line L12 (-43.25, 74.893427) -> (-43.25, 5)
  line L13 (-34.25, 5) -> (-32.75, 5)
  line L14 (-32.75, 5) -> (-32.75, 74.893427)
  line L15 (-32.75, 74.893427) -> (-34.25, 74.893427)
  line L16 (-34.25, 74.893427) -> (-34.25, 5)
  line L17 (-70, 90.006251) -> (-70, 0)
  arc A0 (-70, 90.006251) -> (-15, 90.006251) centre (-42.5, 110) ccw
  line L18 (-15, 0) -> (-15, 90.006251)
  line L19 (-70, 0) -> (-15, 0)
  line L20 (-25.25, 5) -> (-23.75, 5)
  line L21 (-23.75, 5) -> (-23.75, 74.893427)
  line L22 (-23.75, 74.893427) -> (-25.25, 74.893427)
  line L23 (-25.25, 74.893427) -> (-25.25, 5)
  line L24 (-15, 138) -> (-23.212698, 138)
  line L25 (-15, 129.993749) -> (-15, 138)
  arc A1 (-15, 129.993749) -> (-23.212698, 138) centre (-42.5, 110) ccw
  line L26 (-70, 138) -> (-70, 129.993749)
  line L27 (-61.787302, 138) -> (-70, 138)
  arc A2 (-61.787302, 138) -> (-70, 129.993749) centre (-42.5, 110) ccw
  line L28 (-23.212698, 138) -> (-61.787302, 138)
  line L29 (-15, 35) -> (0, 35)
  line L30 (-70, 129.993749) -> (-70, 90.006251)
  line L31 (-15, 90.006251) -> (-15, 129.993749)
  line L32 (-3.4, 0) -> (-11.6, 0)
  point P0 (0, 72)
  constraints: 6 end point, 2 perpendicular, 1 parallel, 1 point on circle
extrude "Extrusion42" cut sketch "Sketch47" against normal blind 4.5 contours L4 L3 L2 L1 | L8 L7 L6 L5 | L12 L11 L10 L9 | L16 L15 L14 L13 | A0 L18 L19 L17 | L30 A2 L28 A1 L31 A0 | L26 L27 A2 | A1 L24 L25 | L23 L22 L21 L20
sketch "Sketch48" plane through (70, -67, -54.5) normal (0, 0, -1) x (-1, 0, 0)
  line L0 (0, 0) -> (55, 0) projected
  line L1 (0, -5) -> (0, 0) projected
  line L2 (55, -5) -> (0, -5) projected
  line L3 (55, 0) -> (55, -5) projected
  point P0 (70, 67)
extrude "Extrusion43" add sketch "Sketch48" along normal up to surface (1.5 mm away)
ref_plane "Work Plane7" through (42.5, 72, 0) normal (0, 0, 1) x (1, 0, 0)
mirror "Mirror6" about plane through (42.5, 72, 0) normal (0, 0, 1) of "Extrusion41", "Extrusion38", "Extrusion37"
sketch "Sketch49" plane through (85, 72, -60.5) normal (0, 0, -1) x (-1, 0, 0)
  line L0 (85, 0) -> (85, -35) projected
  line L1 (0, -35) -> (85, -35)
  line L2 (0, -35) -> (0, -109) projected
  line L3 (85, -109) -> (85, -35) projected
  line L4 (0, -35) -> (85, -35)
  line L5 (85, -35) -> (85, -50)
  line L6 (85, -50) -> (0, -50)
  line L7 (0, -50) -> (0, -35)
  point P0 (85, -72)
  constraints: 10 end point, 2 horizontal, 2 parallel, 1 perpendicular, 1 point on line
extrude "Extrusion44" cut sketch "Sketch49" against normal up to surface (2 mm away)
sketch "Sketch50" plane through (0, 0, 0) normal (-1, 0, 0) x (0, 0, 1)
  line L0 (-58.5, -37) -> (-60.5, -37) projected
  line L1 (-54.5, -66) -> (-54.5, 66) projected
  line L2 (-58.5, -37) -> (-54.5, -37)
  line L3 (-54.5, -37) -> (-54.5, 37)
  line L4 (-54.5, 37) -> (-58.5, 37)
  line L5 (-58.5, 37) -> (-58.5, -37)
  point P0 (0, 0)
  constraints: 8 end point, 2 parallel, 1 coincident, 1 horizontal, 1 perpendicular, 1 point on line
extrude "Extrusion45" cut sketch "Sketch50" against normal blind 2
mirror "Mirror7" about plane through (42.5, 0, 0) normal (1, 0, 0) of "Extrusion45"
mirror "Mirror8" about plane through (42.5, 72, 0) normal (0, 0, 1) of "Extrusion45", "Mirror7"
sketch "Sketch51" plane through (0, 0, 0) normal (-1, 0, 0) x (0, 0, 1)
  line L0 (54.5, -66) -> (-54.5, -66) projected
  line L1 (25.5, -72) -> (-25.5, -72)
  line L2 (-25.5, -72) -> (-25.5, -66)
  line L3 (-25.5, -66) -> (25.5, -66)
  line L4 (25.5, -66) -> (25.5, -72)
  line L5 (-60.5, -72) -> (-60.5, -37) projected
  line L6 (60.5, -37) -> (60.5, -72) projected
  point P0 (0, 0)
  dimension "d268" = 35
  dimension "d269" = 35
  constraints: 8 end point, 2 parallel, 1 horizontal, 1 perpendicular, 1 point on line
  measures "d268" distance between parallel lines of L5 L2
  measures "d269" distance between parallel lines of L6 L4
extrude "Extrusion46" cut sketch "Sketch51" against normal blind 2
sketch "Sketch52" plane through (85, -72, -60.5) normal (0, -1, 0) x (1, 0, 0)
  line L0 (-85, 86) -> (-83, 86) projected
  line L1 (-70, 113) -> (-70, 8) projected
  line L2 (-83, 86) -> (-70, 86)
  line L3 (-70, 86) -> (-70, 35)
  line L4 (-70, 35) -> (-83, 35)
  line L5 (-83, 35) -> (-83, 86)
  point P0 (-85, 60.5)
  constraints: 8 end point, 2 parallel, 1 coincident, 1 horizontal, 1 perpendicular, 1 point on line
extrude "Extrusion47" cut sketch "Sketch52" against normal blind 2
mirror "Mirror9" about plane through (42.5, 0, 0) normal (1, 0, 0) of "Extrusion47", "Extrusion46"
mirror "Mirror10" about plane through (0, 0, 60.5) normal (0, 1, 0) of "Extrusion47", "Extrusion46", "Mirror9"
sketch "Sketch53" plane through (0, -72, -56) normal (0, 0, -1) x (-1, 0, 0)
  circle A0 centre (-42.5, 110) radius 22.5
  circle A1 centre (-42.5, 110) radius 24.5
  circle A2 centre (-25.175884, 127.324116) radius 2
  line L0 (-25.175884, 127.324116) -> (-42.5, 110)
  line L1 (-15, 110) -> (-15, 111.5)
  line L2 (-42.5, 110) -> (-15, 110)
  circle A3 centre (-42.5, 110) radius 21
  circle A4 centre (-25.175884, 127.324116) radius 1
  circle A5 centre (-59.824116, 127.324116) radius 1
  circle A6 centre (-59.824116, 127.324116) radius 2
  circle A7 centre (-59.824116, 92.675884) radius 1
  circle A8 centre (-59.824116, 92.675884) radius 2
  circle A9 centre (-25.175884, 92.675884) radius 1
  circle A10 centre (-25.175884, 92.675884) radius 2
  circle A11 centre (-42.5, 110) radius 23.5
  point P0 (0, 72)
  point P1 (-27.124991, 127.772425)
  point P2 (-57.875009, 127.772425)
  point P3 (-60.272425, 125.375009)
  point P4 (-60.272425, 94.624991)
  point P5 (-57.875009, 92.227575)
  point P6 (-27.124991, 92.227575)
  point P7 (-24.727575, 94.624991)
  point P8 (-24.727575, 125.375009)
  dimension "d274" = 49
  dimension "d275" = 45
  dimension "d276" = 4
  dimension "d277" = 42
  dimension "d278" = 2
  dimension "d281" = 360
  dimension "d283" = 47
  constraints: 10 centre point, 6 coincident, 4 end point, 1 perpendicular, 20 other
  measures "d275" angle of L2 L0
  measures "d276" diameter of A2
  measures "d277" diameter of A3
  measures "d278" diameter of A4
  measures "d283" diameter of A11
extrude "Extrusion48" add sketch "Sketch53" along normal blind 2 contours L2 A11 A10 A0 | A0 A2 A11 L2 | A0 A6 A11 A2 | L0 A11 A2 | A2 A11 L0 | A10 A11 A8 A0 | A10 A11 | A0 A8 A11 A6 | A6 A11 | A2 A1 A4 A11 | A11 A4 A1 A2 | A8 A11 | A10 A1 A9 A11 | A11 A9 A1 A10 | A6 A1 A5 A11 | A2 A1 A4 | A11 A5 A1 A6 | A11 A7 A1 A8 | A10 A1 A9 | A8 A1 A7 A11 | A6 A1 A5 | A1 A7 A8
sketch "Sketch54" plane through (42.5, 38, -56) normal (0, 0, -1) x (-1, 0, 0)
  circle A0 centre (0, 0) radius 3 projected
  circle A1 centre (0, 0) radius 20
  point P0 (42.5, -38)
  dimension "d286" = 40
  constraints: 1 centre point, 1 coincident
  measures "d286" diameter of A1
extrude "Extrusion49" add sketch "Sketch54" along normal blind 1 contours A0 | A1
sketch "Sketch55" plane through (42.5, 38, -57) normal (0, 0, -1) x (-1, 0, 0)
  circle A0 centre (0, 0) radius 3 projected
  circle A1 centre (0, 0) radius 15
  point P0 (42.5, -38)
  dimension "d289" = 30
  constraints: 1 centre point, 1 coincident
  measures "d289" diameter of A1
extrude "Extrusion50" add sketch "Sketch55" along normal blind 1 contours A0 | A1
sketch "Sketch56" plane through (85, 72, -60.5) normal (0, 0, -1) x (-1, 0, 0)
  circle A0 centre (77, -124) radius 4.1 projected
  circle A1 centre (7, -124) radius 4.1 projected
  circle A2 centre (7, -20) radius 4.1
  circle A3 centre (77, -20) radius 4.1
  line L0 (85, 0) -> (0, 0) projected
  point P0 (85, -72)
  dimension "d292" = 20
  constraints: 2 centre point, 2 equal radius, 2 vertical alignment, 1 horizontal alignment
  measures "d292" distance from line of A3.centre L0
extrude "Extrusion51" cut sketch "Sketch56" against normal blind 6
ref_plane "Work Plane8" through (42.5, 44.5, 74) normal (0, 1, 0) x (-1, 0, 0)
sketch "Sketch57" plane through (42.5, 44.5, 74) normal (0, 1, 0) x (-1, 0, 0)
  line L0 (6.5, 25) -> (-6.5, 25) projected
  line L1 (-6.5, 0) -> (6.5, 0) projected
  line L2 (-0.5, 0) -> (-0.5, 0)
  line L3 (-3, 2.5) -> (-3, 17.5)
  line L4 (-0.5, 20) -> (-0.5, 20)
  line L5 (2, 17.5) -> (2, 2.5)
  arc A0 (-0.5, 0) -> (2, 2.5) centre (-0.5, 2.5) ccw
  arc A1 (-3, 2.5) -> (-0.5, 0) centre (-0.5, 2.5) ccw
  arc A2 (2, 17.5) -> (-0.5, 20) centre (-0.5, 17.5) ccw
  arc A3 (-0.5, 20) -> (-3, 17.5) centre (-0.5, 17.5) ccw
  point P0 (42.5, -74)
  point P1 (-3, 20)
  point P2 (-3, 0)
  point P3 (2, 20)
  point P4 (-0.5, 0)
  point P5 (-0.5, 20)
  dimension "d295" = 4.5
  dimension "d296" = 5
  dimension "d297" = 20
  dimension "d298" = 5
  dimension "d299" = 2.5
  dimension "d300" = 2.5
  constraints: 8 end point, 8 point on circle, 8 tangent, 6 point on line, 4 centre point, 2 concentric, 2 parallel, 1 horizontal, 1 perpendicular
  measures "d295" distance from line of L0.start L5
  measures "d296" distance of point (-3, 20) point (2, 20)
  measures "d297" distance of point (-3, 0) point (-3, 20)
  measures "d298" distance between parallel lines of L0 L4
  measures "d299" radius of A0
  measures "d300" radius of A2
extrude "Extrusion52" [suppressed]
sketch "Sketch58" plane through (84, -12, 0) normal (1, 0, 0) x (0, 0, -1)
  circle A0 centre (0, 0) radius 20
  circle A1 centre (0, 0) radius 35
  circle A2 centre (0, 0) radius 12.5
  line L0 (-4, 15.8) -> (4, 15.8)
  line L1 (-4, 15.8) -> (-4, 11.842719)
  line L2 (4, 15.8) -> (4, 11.842719)
  point P0 (0, 12)
  dimension "d305" = 25
  dimension "d306" = 15.8
  dimension "d307" = 8
  dimension "d308" = 4
  constraints: 6 end point, 2 point on circle, 1 centre point, 1 coincident, 1 horizontal, 1 parallel, 1 vertical
  measures "d305" diameter of A2
  measures "d306" distance from line of A0.centre L0
  measures "d307" distance of L0.start L0.end
  measures "d308" horizontal distance of point (0, 12) L0.end
extrude "Extrusion53" [suppressed]
sketch "Sketch59" plane through (86, -12, 0) normal (1, 0, 0) x (0, 0, -1)
  circle A0 centre (0, 0) radius 20
  line L0 (4, 15.8) -> (4, 11.842719)
  arc A1 (-4, 11.842719) -> (4, 11.842719) centre (0, 0) ccw
  line L1 (-4, 11.842719) -> (-4, 15.8)
  line L2 (-4, 15.8) -> (4, 15.8)
  point P0 (0, 12)
extrude "Extrusion54" [suppressed]
thread "Thread11" size "M6x1" class "6H" standard "ANSI Metric M Profile" length 60
chamfer "Chamfer1" distance 0.5 angle 45 1 edges at (36, 38, 99)
chamfer "Chamfer2" [suppressed]
body "Solid1"
